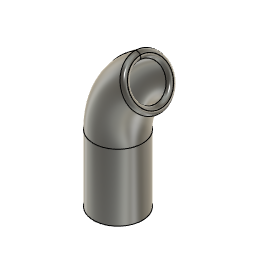
filter-outflow (Autodesk Fusion 360 design; units mm, degrees)
Autodesk Fusion 360 part; units mm, degrees
sketch "Sketch1" plane through (0, 0, 0) normal (0, 0, 1) x (1, 0, 0)
  circle A0 centre (0, 0) radius 9
  circle A1 centre (0, 0) radius 11
  dimension "d1" = 18
  dimension "d2" = 2
  constraint coincident A0.centre A1.centre
  measures "d1" diameter of A0
extrude "Extrude1" add sketch "Sketch1" along normal blind 30
draft "Draft1" angle 2.6 neutral plane through (0, 0, 0) pull (0, 0, -1) 1 faces at (8.9553, -0.8961, 20)
sketch "Sketch2" plane through (0, 0, 0) normal (0, 1, 0) x (1, 0, 0)
  arc A0 (0, -30) -> (30, -60) centre (29.5, -30.5) ccw
sweep "Sweep1" add 1 faces at (9.8098, -0.9259, 30) path "Sketch2" along A0 for 0.66 of its length starting at (0, 0, 30) heading (-0.0169, 0, 0.9999)
fillet "Fillet1" radius 1.669 2 edges at (9.5973, -3.9778, 64.9186) (11.1323, 2.7619, 62.1854)
